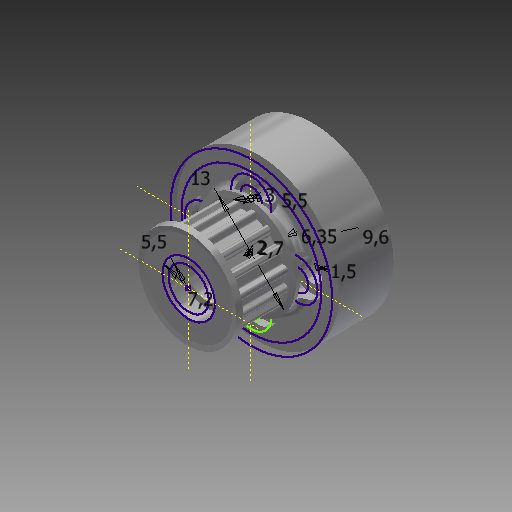
# Autodesk Inventor part: Synchrone Riemenscheibe1
Saved by Autodesk Inventor 2018.3 (Build 223284000, 284)
## iProperties
Created: 2018-07-27
Part Number: Synchrone Riemenscheibe1
Material: Steel
Document SubType Name: Modeling
Designer: JochenAlt
Density: 1 g/cm^3
Appearance: Steel
CustomPartVersion: 1
Author: JochenAlt
Autodesk Inventor part; units mm, degrees
ref_plane "YZ Plane" through (0, 0, 0) normal (1, 0, 0) x (0, 1, 0)
ref_plane "XZ Plane" through (0, 0, 0) normal (0, 1, 0) x (-1, 0, 0)
ref_plane "XY Plane" through (0, 0, 0) normal (0, 0, 1) x (1, 0, 0)
sketch "Riemenscheibenskizze" plane through (0, 0, 0) normal (0, 0, 1) x (1, 0, 0)
  circle A0 centre (0, 0) radius 6.3662 construction
  circle A1 centre (0, 0) radius 6.0662
  circle A2 centre (0, 0) radius 5.3162
  line L0 (-0.847, 6.0068) -> (-0.525, 5.3162)
  line L1 (-0.525, 5.3162) -> (0.525, 5.3162)
  line L2 (0.525, 5.3162) -> (0.847, 6.0068)
  line L3 (0, 0) -> (0, 6.0662) construction
  point P0 (0, 5.3162)
  dimension "d0" = 12.7324
  dimension "d1" = 0.3
  dimension "d2" = 0.75
  dimension "d3" = 50
  dimension "d4" = 1.05
  constraints: 8 end point, 3 coincident, 3 point on circle, 2 centre point, 1 horizontal, 1 midpoint, 1 point on line, 1 vertical, 1 vertical alignment, 3 other
  measures "d0" diameter of A0
  measures "d1" radial gap between concentric circles of A0 A1
  measures "d3" angle of L2 L0
  measures "d4" distance of L0.end L1.end
extrude "Grundkörper" add sketch "Riemenscheibenskizze" along normal mid plane 7 contours A2 | A1 L0 L1 L2 | L2 L1 L0 A1
extrude "Zahn" cut sketch "Riemenscheibenskizze" along normal through all both and the other way through all contours L2 L1 L0 A1 picked at (0, 5.8118)
fillet "Fillet" radius 0.2 2 edges at (0.525, 5.3162, 0) (-0.525, 5.3162, 0)
fillet "Fillet" radius 0.3 4 edges at (-0.847, 6.0068, 1.75) (-0.847, 6.0068, -1.75) (0.847, 6.0068, 1.75) (0.847, 6.0068, -1.75)
pattern_circular "Zähne" count 16 over 360 about axis through (0, 0, -10) along (0, 0, 1) of "Zahn", "Fillet"
pulley flange "Flansch links" diameter 12.1324 height 0.8 thickness 0.8 bend angle 10 centre (0, 0, -3.5) toward (0, 0, -1)
pulley flange "Flansch rechts" diameter 12.1324 height 0.8 thickness 0.8 bend angle 10 centre (0, 0, 3.5) toward (0, 0, 1)
sketch "Skizze2" plane through (0, 0, -4.3) normal (0, 0, 1) x (1, 0, 0)
  line L0 (-15.54, 0) -> (15.54, 0) construction
  circle A0 centre (0, 0) radius 9.6
  circle A1 centre (0, 0) radius 11.1
  circle A2 centre (0, 0) radius 6.35 construction
  line L1 (0, 15.54) -> (0, -15.54) construction
  circle A3 centre (0, 6.35) radius 1.5
  circle A4 centre (6.35, 0) radius 1.5
  circle A5 centre (0, -6.35) radius 1.5
  circle A6 centre (-6.35, 0) radius 1.5
  circle A7 centre (0, 0) radius 1
  circle A8 centre (0, 6.35) radius 2.75
  circle A9 centre (6.35, 0) radius 2.75
  circle A10 centre (0, -6.35) radius 2.75
  circle A11 centre (-6.35, 0) radius 2.75
  circle A12 centre (0, 0) radius 1.35 construction
  line L2 (0.7794, 1.35) -> (1.5588, 0)
  line L3 (1.5588, 0) -> (0.7794, -1.35)
  line L4 (0.7794, -1.35) -> (-0.7794, -1.35)
  line L5 (-0.7794, -1.35) -> (-1.5588, 0)
  line L6 (-1.5588, 0) -> (-0.7794, 1.35)
  line L7 (-0.7794, 1.35) -> (0.7794, 1.35)
  circle A13 centre (0, 0) radius 6.5
  point P0 (0, 0)
  point P1 (0, 1.35)
  dimension "d26" = 2.7
  dimension "d18" = 9.6
  dimension "d19" = 1.5
  dimension "d20" = 6.35
  dimension "d21" = 3
  dimension "d23" = 2
  dimension "d27" = 5.5
  dimension "d48" = 13
  constraints: 13 centre point, 12 end point, 11 coincident, 6 equal radius, 4 point on circle, 4 point on line, 1 midpoint, 1 vertical alignment, 15 other
  measures "d18" radius of A0
  measures "d19" radial gap between concentric circles of A1 A0
  measures "d20" radius of A2
  measures "d21" diameter of A3
  measures "d23" diameter of A7
  measures "d27" diameter of A8
  measures "d48" diameter of A13
extrude "Extrusion3" add sketch "Skizze2" against normal blind 1 separate body contours A13 A3 | A3 A13 A8 | A8 A13 A9 A10 A11 | A11 A13 A6 | A13 A4 A9 | A6 A13 | A13 A4 | A10 A13 A5 | A5 A13 | L2 L3 L4 L5 L6 L7 picked at (-0.0596, 5.9405) picked at (2.0583, 5.6656) picked at (-5.6808, 2.0662) picked at (5.6656, -2.0583) picked at (-5.937, 0) picked at (5.9753, -0.3435) picked at (2.0583, -5.6656) picked at (-0.0596, -5.9405)
extrude "Extrusion12" add sketch "Skizze2" against normal blind 2.5 from surface at -1 contours A0 | A1 | A3 A13 | A3 A13 A8 | A13 A3 | A3 A13 A8 | A8 A13 A9 A10 A11 | A13 A6 A11 | A11 A13 A6 | A13 A4 A9 | A9 A13 A4 | A13 A6 | A6 A13 | A13 A4 | A4 A13 | A13 A5 A10 | A10 A13 A5 | A13 A5 | A5 A13 | L2 L3 L4 L5 L6 L7 bodies 2
extrude "Extrusion14" cut sketch "Skizze2" against normal through all contours A3 A13 | A13 A3 | A13 A6 | A6 A13 | A13 A4 | A4 A13 | A13 A5 | A5 A13 bodies 2
extrude "Extrusion4" cut sketch "Skizze2" against normal blind 2 from surface at 0 contours A3 A13 | A3 A13 A8 | A13 A3 | A3 A13 A8 | A13 A6 A11 | A11 A13 A6 | A13 A4 A9 | A9 A13 A4 | A13 A6 | A6 A13 | A13 A4 | A4 A13 | A13 A5 A10 | A10 A13 A5 | A13 A5 | A5 A13 bodies 1 2
extrude "Extrusion6" cut sketch "Skizze2" along normal through all contours A7 bodies 1
sketch "Skizze3" plane through (0, 0, 4.3) normal (0, 0, 1) x (1, 0, 0)
  line L0 (0, 9.6127) -> (0, -9.6127) construction
  line L1 (-9.6127, 0) -> (9.6127, 0) construction
  circle A0 centre (0, 0) radius 2.75
  circle A1 centre (0, 0) radius 3.6
  point P0 (0, 0)
  dimension "d43" = 5.5
  dimension "d60" = 7.2
  constraints: 2 centre point, 2 coincident
  measures "d43" diameter of A0
  measures "d60" diameter of A1
extrude "Extrusion10" cut sketch "Skizze3" against normal blind 5 contours A0 bodies 1
extrude "Extrusion9" add sketch "Skizze2" against normal blind 5 from surface at -3.5 contours A1 bodies 2
extrude "Extrusion13" cut sketch "Skizze2" along normal blind 1.8 from surface at -3.5 contours L2 L3 L4 L5 L6 L7 bodies 2
fillet "Rundung3" radius 1 4 edges at (4.5962, 4.5962, -5.3) (4.5962, -4.5962, -5.3) (-4.5962, -4.5962, -5.3) (-4.5962, 4.5962, -5.3)
extrude "Extrusion15" cut sketch "Skizze3" against normal blind 2.5 bodies 1
equation "\"d1\" = da_a"
equation "\"d2\" = da_hg"
equation "\"d3\" = 2 * da_fi"
equation "\"d4\" = da_bw"
equation "\"d5\" = da_bf"
equation "\"d7\" = da_bf"
equation "\"d9\" = da_rb"
equation "\"d10\" = da_rt"
equation "\"da_pb\" = 2.5"
equation "\"da_fi\" = 25deg"
equation "\"da_hg\" = 0.75"
equation "\"da_bw\" = 1.05"
equation "\"da_rb\" = 0.2"
equation "\"da_rt\" = 0.3"
equation "\"da_a\" = 0.3"
equation "\"da_bf\" = 7"
equation "\"da_wf\" = 0.8"
equation "\"da_hf\" = 0.8"
body "Solid1"
